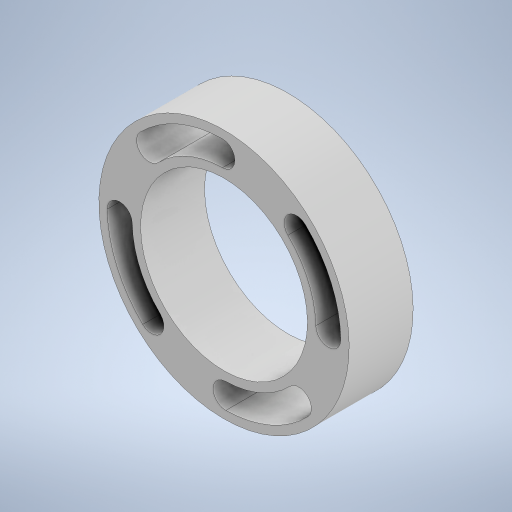
# Autodesk Inventor part: Loose Clutch
Saved by Autodesk Inventor 2024.3 (Build 283343000, 343)
## iProperties
Created: 2024-11-08
Part Number: Loose Clutch
Material: Generic
Document SubType Name: Modeling
Designer: wszaf
Density: 1 g/cm^3
Appearance: Default
Author: wszaf
Autodesk Inventor part; units mm, degrees
ref_plane "YZ Plane" through (0, 0, 0) normal (1, 0, 0) x (0, 1, 0)
ref_plane "XZ Plane" through (0, 0, 0) normal (0, 1, 0) x (-1, 0, 0)
ref_plane "XY Plane" through (0, 0, 0) normal (0, 0, 1) x (1, 0, 0)
sketch "Sketch1" plane through (11.3318, -11.7902, 0) normal (0, 0, 1) x (0.9999, 0.0157, 0)
  circle A0 centre (0, 0) radius 6
  circle A1 centre (0, 0) radius 9
  arc A2 (7.5, 0) -> (5.3033, 5.3033) centre (0, 0) ccw construction
  arc A3 (9, 0) -> (6.364, 6.364) centre (0, 0) ccw
  arc A4 (6, 0) -> (4.2426, 4.2426) centre (0, 0) ccw
  arc A5 (6, 0) -> (9, 0) centre (7.5, 0) ccw
  arc A6 (6.364, 6.364) -> (4.2426, 4.2426) centre (5.3033, 5.3033) ccw
  line L0 (0, 0) -> (5.3033, 5.3033) construction
  line L1 (0, 0) -> (7.5, 0) construction
  arc A7 (6.6, 0) -> (4.6669, 4.6669) centre (0, 0) ccw
  arc A8 (6.6, 0) -> (8.4, 0) centre (7.5, 0) ccw
  arc A9 (8.4, 0) -> (5.9397, 5.9397) centre (0, 0) ccw
  arc A10 (5.9397, 5.9397) -> (4.6669, 4.6669) centre (5.3033, 5.3033) ccw
  point P0 (-11.1453, 11.9666)
  dimension "d0" = 12
  dimension "d8" = 18
  dimension "d9" = 45
  dimension "d10" = 1.5
  dimension "d12" = 0.6
  dimension "d15" = 7.5
  constraints: 18 point on circle, 11 centre point, 4 end point, 4 tangent, 2 coincident, 1 horizontal alignment, 4 other
  measures "d0" diameter of A0
  measures "d8" diameter of A1
  measures "d9" angle of L1 L0
  measures "d10" radius of A5
  measures "d12" radial gap between concentric circles of A6 A10
  measures "d15" distance of A0.centre L1.end
extrude "Extrusion1" add sketch "Sketch1" along normal blind 4.6 contours A5 A1 A6 A0 | A0 A6 A1 A5 | A7 A10 A9 A8
extrude "Extrusion2" cut sketch "Sketch1" along normal blind 4.6 contours A7 A10 A9 A8
pattern_circular "Circular Pattern1" count 4 over 360 about axis through (11.3318, -11.7902, 0) along (0, 0, 1) of "Extrusion2"
equation "\"d15\" = 0.25 * d0 + 0.25 * d8"
equation "\"d13\" = Clutch_Width - Fit_Loose"
equation "\"d16\" = Clutch_Width - Fit_Loose"
equation "\"Clutch_Width\" = 5"
equation "\"Fit_Loose\" = 0.4"
body "Solid1"
